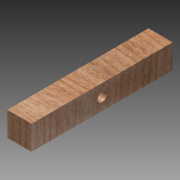
# Autodesk Inventor part: CNC-1.1v-X-7-( axis mover nut inside)
Saved by Autodesk Inventor 2015 (Build 190159000, 159)
## iProperties
Created: 2015-07-14
Part Number: CNC-1.1v-X-7-( axis mover nut inside)
Material: Generic
Document SubType Name: Modeling
Designer: Bangladesh
Density: 1 g/cm^3
Appearance: Default
Author: Bangladesh
Autodesk Inventor part; units mm, degrees
ref_plane "YZ Plane" through (0, 0, 0) normal (1, 0, 0) x (0, 1, 0)
ref_plane "XZ Plane" through (0, 0, 0) normal (0, 1, 0) x (-1, 0, 0)
ref_plane "XY Plane" through (0, 0, 0) normal (0, 0, 1) x (1, 0, 0)
sketch "Sketch1" plane through (0, 0, 0) normal (0, 1, 0) x (-1, 0, 0)
  line L0 (19.05, 111.1) -> (-19.05, 111.1)
  line L1 (-19.05, 111.1) -> (-19.05, -111.1)
  line L2 (-19.05, -111.1) -> (19.05, -111.1)
  line L3 (19.05, -111.1) -> (19.05, 111.1)
  line L4 (19.05, 111.1) -> (-19.05, -111.1) construction
  line L5 (-19.05, 111.1) -> (19.05, -111.1) construction
  point P0 (0, 0)
  dimension "d0" = 222.2
  dimension "d1" = 38.1
  constraints: 12 end point, 2 midpoint, 2 parallel, 1 horizontal, 1 perpendicular
  measures "d0" distance of L2.end L0.start
  measures "d1" distance of L1.end L2.end
extrude "Extrusion1" add sketch "Sketch1" along normal mid plane 38.1
sketch "Sketch2" plane through (19.05, -19.05, -111.1) normal (1, 0, 0) x (0, 0, -1)
  circle A0 centre (-111.1, 19.05) radius 7.15
  point P0 (-111.1, 11.9)
  dimension "d4" = 14.3
  constraints: 2 coincident, 1 vertical alignment, 2 other
extrude "Extrusion2" cut sketch "Sketch2" against normal through all
body "Solid1"
